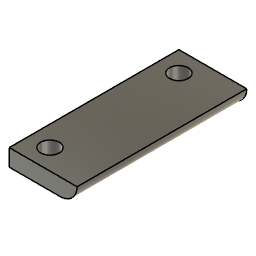
Pipette holder clamp v11 (Autodesk Fusion 360 design; units mm, degrees)
Autodesk Fusion 360 part; units mm, degrees
note: some values were not read from the file. Set by a fixed rule: which sketch regions a step uses.
sketch "Sketch3" plane through (0, 0, 0) normal (0, 0, 1) x (1, 0, 0)
  line L0 (0, 0) -> (20, 0)
  line L1 (20, 0) -> (20, 50)
  line L2 (20, 50) -> (0, 50)
  line L3 (0, 50) -> (0, 0)
  dimension "d19" = 20
  dimension "d20" = 50
  constraint horizontal L0
  constraint vertical L1
  constraint horizontal L2
  constraint vertical L3
  constraint coincident L0.start L3.end
  measures "d19" distance of L0.start L0.end
  measures "d20" distance of L0.start L2.end
extrude "Extrude1" add sketch "Sketch3" along normal blind 5
fillet "Fillet2" radius 5 1 edges at (20, 25, 0)
sketch "Sketch7" plane through (0, 0, 5) normal (0, 0, 1) x (-1, 0, 0)
  line L0 (0, -50) -> (0, 0)
  line L1 (0, 0) -> (-20, 0)
  line L2 (-20, 0) -> (-20, -50)
  line L3 (-20, -50) -> (0, -50)
  circle A0 centre (-6, -6) radius 2.75
  circle A1 centre (-6, -44) radius 2.75
  dimension "d47" = 5.5
  dimension "d48" = 5.5
  dimension "d49" = 6
  dimension "d50" = 6
  dimension "d51" = 6
  dimension "d52" = 6
  measures "d47" diameter of A0
  measures "d48" diameter of A1
  measures "d49" distance of L1 A0.centre
  measures "d50" distance of L0 A0.centre
  measures "d51" distance of L0 A1.centre
  measures "d52" distance of L3 A1.centre
extrude "Extrude5" cut sketch "Sketch7" against normal blind 5 contours A0 | A1
